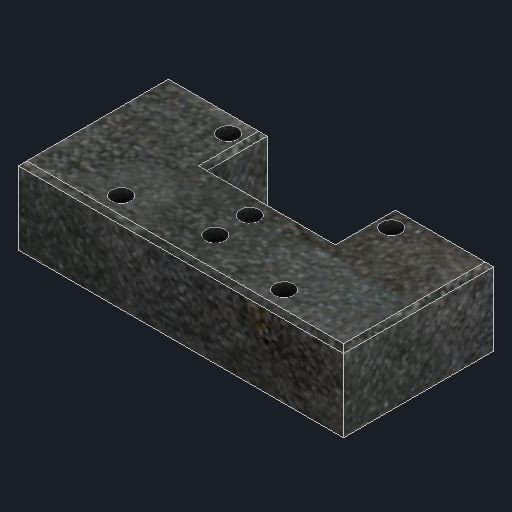
# Autodesk Inventor part: GROUNDPLATE PART 1
Saved by Autodesk Inventor 2023 (Build 270158000, 158)
## iProperties
Created: 2020-07-01
Part Number: GROUNDPLATE PART 1
Material: Steel ASTM A36
Document SubType Name: Modeling
Designer: Smit Ambardekar
Density: 7.85 g/cm^3
Appearance: Plate
Author: Smit Ambardekar
Autodesk Inventor part; units mm, degrees
ref_plane "YZ Plane" through (0, 0, 0) normal (1, 0, 0) x (0, 1, 0)
ref_plane "XZ Plane" through (0, 0, 0) normal (0, 1, 0) x (-1, 0, 0)
ref_plane "XY Plane" through (0, 0, 0) normal (0, 0, 1) x (1, 0, 0)
sketch "Sketch1" plane through (0, 0, 0) normal (0, 1, 0) x (-1, 0, 0)
  line L0 (37.9, -17.5) -> (37.9, 17.5)
  line L1 (37.9, 17.5) -> (-37.9, 17.5)
  line L2 (-37.9, 17.5) -> (-37.9, -17.5)
  line L3 (37.9, -17.5) -> (14.9, -17.5)
  line L4 (14.9, -17.5) -> (14.9, -3.5)
  line L5 (14.9, -3.5) -> (-15, -3.5)
  line L6 (-15, -3.5) -> (-15, -17.5)
  line L7 (-37.9, -17.5) -> (-15, -17.5)
  line L8 (14.9, -17.5) -> (37.9, -17.5)
  circle A0 centre (-0.019, 9.5) radius 2.25
  circle A1 centre (-0.0381, 1.5) radius 2.25
  circle A2 centre (18.9586, -12.5) radius 2.25
  circle A3 centre (-19.0414, -12.5) radius 2.25
  circle A4 centre (-19.0414, 12.5) radius 2.25
  circle A5 centre (18.9586, 12.5) radius 2.25
  line L9 (18.9586, -12.5) -> (-19.0414, -12.5)
  line L10 (5.1, -12.5) -> (-13.9, -12.5)
  point P0 (0, 0)
  dimension "d0" = 75.8
  dimension "d1" = 35
  dimension "d2" = 23
  dimension "d3" = 14
  dimension "d4" = 29.9
  dimension "d7" = 4.5
  dimension "d8" = 4.5
  dimension "d11" = 4.5
  dimension "d12" = 4.5
  dimension "d20" = 38
  dimension "d21" = 0
  dimension "d23" = 38
  constraints: 22 end point, 6 centre point, 6 perpendicular, 3 horizontal, 3 parallel
  measures "d0" distance of L1.end L0.end
  measures "d1" distance of L0.end L0.start
  measures "d2" distance of L0.start L3.end
  measures "d3" distance of L3.end L4.end
  measures "d4" distance of L4.end L5.end
  measures "d7" diameter of A0
  measures "d8" diameter of A1
  measures "d11" diameter of A2
  measures "d12" diameter of A3
  measures "d20" distance of L9.end L9.start
  measures "d21" horizontal distance of A5.centre L9.start
  measures "d23" distance of A4.centre A5.centre
extrude "Extrusion1" add sketch "Sketch1" along normal blind 18 contours L3 L4 L5 L6 L7 L2 L1 L0
chamfer "Chamfer1" distance 1 angle 45 8 edges at (-37.9, 18, 0) (0, 18, 17.5) (37.9, 18, 0) (-26.4, 18, -17.5) (26.45, 18, -17.5) (-14.9, 18, -10.5) (0.05, 18, -3.5) (15, 18, -10.5)
body "Solid1"
